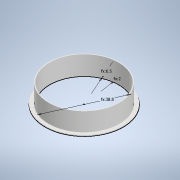
# Autodesk Inventor part: tpuBase
Saved by Autodesk Inventor 2022 (Build 260153000, 153)
## iProperties
Created: 2023-05-09
Part Number: tpuBase
Material: Generic
Document SubType Name: Modeling
Designer: Hallgato
Density: 1 g/cm^3
Appearance: Default
Author: Hallgato
Autodesk Inventor part; units mm, degrees
ref_plane "YZ Plane" through (0, 0, 0) normal (1, 0, 0) x (0, 1, 0)
ref_plane "XZ Plane" through (0, 0, 0) normal (0, 1, 0) x (-1, 0, 0)
ref_plane "XY Plane" through (0, 0, 0) normal (0, 0, 1) x (1, 0, 0)
sketch "Sketch1" plane through (0, 0, 0) normal (0, 1, 0) x (-1, 0, 0)
  circle A0 centre (0, 0) radius 19.4
  circle A1 centre (0, 0) radius 18.9
  circle A2 centre (0, 0) radius 21.4
  dimension "d0" = 38.8
  dimension "d1" = 0.5
  dimension "d4" = 2
  constraints: 3 centre point, 3 coincident
  measures "d0" diameter of A0
  measures "d1" radial gap between concentric circles of A0 A1
  measures "d4" radial gap between concentric circles of A2 A0
extrude "Extrusion1" add sketch "Sketch1" along normal blind 10.5 contours A0
extrude "Extrusion2" add sketch "Sketch1" along normal blind 0.5 contours A2
equation "\"d0\" = bottleDiameter"
equation "\"d1\" = tpuTick"
equation "\"d4\" = 4 * tpuTick"
equation "\"d5\" = tpuTick"
equation "\"capDiameter\" = 29.5"
equation "\"bottleLen\" = 81.3"
equation "\"bottleDiameter\" = 38.8"
equation "\"tubeInsideDiameter\" = 2"
equation "\"tubeOutsideDiameter\" = 5.4"
equation "\"tick\" = 2"
equation "\"connectorDiameter\" = 35"
equation "\"connectorInsideDiameter\" = tubeInsideDiameter - tick"
equation "\"connectorTubeDepth\" = 18.5"
equation "\"tubeFlapDepth\" = 3"
equation "\"tubeFlapAngle\" = 15deg"
equation "\"minTick\" = 0.25"
equation "\"tubeLinkTick\" = 2"
equation "\"tubeTolerance\" = 0.3"
equation "\"tickHolder\" = 1"
equation "\"tpuTick\" = 0.5"
body "Solid1"
